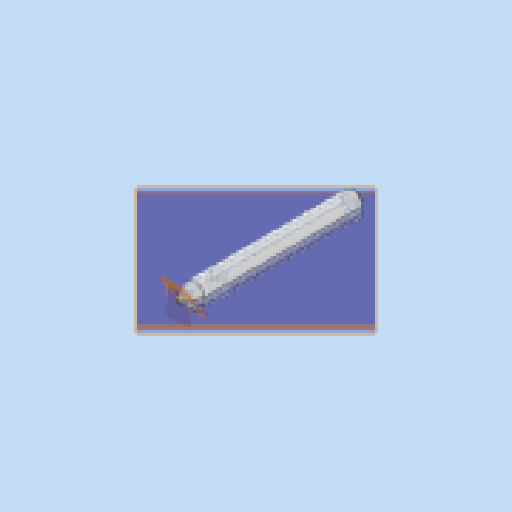
# Autodesk Inventor part: Shell
Saved by Autodesk Inventor 2024 (Build 280153000, 153)
## iProperties
Created: 2025-03-21
Part Number: Shell
Material: Generic
Document SubType Name: Modeling
Designer: XxPan
Density: 1 g/cm^3
Appearance: Default
Author: XxPan
Autodesk Inventor part; units mm, degrees
ref_plane "YZ Plane" through (0, 0, 0) normal (1, 0, 0) x (0, 1, 0)
ref_plane "XZ Plane" through (0, 0, 0) normal (0, 1, 0) x (-1, 0, 0)
sketch "Sketch1" plane through (0, 0, 0) normal (0, 0, 1) x (1, 0, 0)
  line L0 (0, 0) -> (0, -6) construction
  line L1 (-9, 0) -> (-9, -6)
  line L2 (9, -6) -> (9, 0)
  arc A0 (9, 0) -> (-9, 0) centre (0, 0) ccw
  arc A1 (-9, -6) -> (9, -6) centre (0, -6) ccw
  point P0 (0, -3)
  dimension "d0" = 6
  dimension "d1" = 18
  constraints: 8 end point, 4 point on circle, 4 tangent, 2 centre point, 1 midpoint, 1 parallel, 1 vertical
  measures "d0" distance of L0.start L0.end
  measures "d1" diameter of A1
extrude "Extrusion1" add sketch "Sketch1" against normal blind 150
chamfer "Chamfer1" distance 2 angle 45 4 edges at (0, 9, -150) (9, -3, -150) (0, -15, -150) (-9, -3, -150)
shell "Shell1" thickness 1 removed faces 1 at (1.0638, -8.805, 0)
ref_plane "Work Plane1" through (0, 0, 15) normal (0, 0, 1) x (1, 0, 0)
sketch "Sketch2" plane through (0, 0, 15) normal (0, 0, 1) x (1, 0, 0)
  circle A0 centre (0, 0) radius 2
  dimension "d3" = 4
  constraints: 1 centre point, 1 coincident
  measures "d3" diameter of A0
loft "Loft1" add profiles "Sketch1", "Sketch2" separate body
sketch "Sketch3" plane through (0, 0, 15) normal (0, 0, 1) x (1, 0, 0)
  circle A0 centre (0, 0) radius 0.6
  dimension "d14" = 1.2
  constraints: 1 centre point, 1 coincident
  measures "d14" diameter of A0
ref_plane "Work Plane2" through (-8.2598, -14.025, 0) normal (0, 0, 1) x (1, 0, 0)
extrude "Extrusion2" cut sketch "Sketch3" against normal up to surface (15 mm away) bodies 2
sketch "Sketch4" plane through (0, 0, 0) normal (1, 0, 0) x (0, 1, 0)
  line L0 (-6, 0) -> (-15, 0) projected
  line L1 (-15, 0) -> (14.5608, 20.6987)
  line L2 (-15, 0) -> (21.0871, 0) construction
  point P0 (0, 0)
  dimension "d17" = 35
  constraints: 4 end point, 1 equal length, 1 horizontal
  measures "d17" angle of L2 L1
surface extrude "ExtrusionSrf1" sketch "Sketch4" along normal mid plane 20 shown yes curves L1
sketch "Sketch5" plane through (0, 0, 15) normal (0, 0, 1) x (1, 0, 0)
  circle A0 centre (0, -7) radius 4
  line L0 (0, -18) -> (0, 3) construction
  line L1 (10, -15) -> (-10, -15) projected
  line L2 (-4, -7) -> (-4, -15)
  line L3 (4, -7) -> (4, -15)
  point P0 (0, 0)
  dimension "d20" = 8
  dimension "d21" = 8
  constraints: 4 end point, 3 point on line, 2 perpendicular, 2 point on circle, 2 tangent, 1 centre point
  measures "d20" diameter of A0
  measures "d21" distance from line of L1 A0.centre
extrude "Extrusion3" cut sketch "Sketch5" against normal up to surface surface through (0, -15, 0) normal (0, 0.5735764, -0.819152) bodies 2
ref_plane "Work Plane4" through (-10, 15.7079, 19.0604) normal (0, -0.5735764, 0.819152) x (1, 0, 0)
sketch "Sketch6" plane through (0, 0, 0) normal (0, 0, 1) x (1, 0, 0)
  arc A0 (4, -7) -> (-4, -7) centre (0, -7) ccw projected
  circle A1 centre (0, -7) radius 4
  point P0 (0, 0)
  point P1 (4, -7)
  constraints: 1 coincident, 3 other
extrude "Extrusion4" cut sketch "Sketch6" along normal up to surface surface through (0, -15, 0) normal (0, 0.5735764, -0.819152) bodies 2
sketch "Sketch7" plane through (4, -12.3169, 1.8787) normal (0, -0.5735764, 0.819152) x (1, 0, 0)
  line L0 (-4, 7.3739) -> (-4, 3.3739) construction
  line L1 (-8, 7.3739) -> (-8, 3.3739)
  line L2 (0, 3.3739) -> (0, 7.3739)
  arc A0 (0, 7.3739) -> (-8, 7.3739) centre (-4, 7.3739) ccw
  arc A1 (-8, 3.3739) -> (0, 3.3739) centre (-4, 3.3739) ccw
  line L3 (0, 0) -> (0, 6.4908) projected
  ellipse E0 centre (-4, 6.4908) end of major axis (-4, 1.6077) minor radius 4 (0, 6.4908) -> (-8, 6.4908) ccw projected
  point P0 (-4, 9.0119)
  point P1 (-4, 5.3739)
  point P2 (0, 6.4908)
  dimension "d27" = 4
  dimension "d28" = 8
  constraints: 8 end point, 4 point on circle, 4 tangent, 2 centre point, 1 collinear, 1 midpoint, 1 parallel, 1 vertical, 2 other
  measures "d27" distance of L0.start L0.end
  measures "d28" diameter of A1
extrude "Extrusion5" cut sketch "Sketch7" along normal blind 1 and the other way blind 1 contours E0 L2 A1 L1 bodies 2
ref_plane "Work Plane5" through (5, -1.8, -20.16) normal (0, 0, -1) x (-1, 0, 0)
sketch "Sketch8" plane through (5, -1.8, -20.16) normal (0, 0, -1) x (-1, 0, 0)
  arc A0 (13, 1.8) -> (-3, 1.8) centre (5, 1.8) ccw projected
  line L0 (-3, 1.8) -> (-3, -4.2) projected
  line L1 (13, -4.2) -> (13, 1.8) projected
  arc A1 (-3, -4.2) -> (13, -4.2) centre (5, -4.2) ccw projected
  line L2 (-1, 7.0915) -> (-1, -4.2)
  line L3 (-3, -4.2) -> (-1, -2.2)
  line L4 (-3, -4.2) -> (-0.1716, -4.2) construction
  dimension "d33" = 2
  dimension "d34" = 45
  constraints: 6 end point, 1 equal length, 1 horizontal, 1 parallel, 1 point on circle, 1 point on line
  measures "d33" distance between parallel lines of L0 L2
  measures "d34" angle of L4 L3
extrude "Extrusion6" add sketch "Sketch8" along normal blind 3 contours L1 A1 L3 L2 A0 bodies 1
sketch "Sketch9" plane through (5, -1.8, -20.16) normal (0, 0, 1) x (1, 0, 0)
  circle A0 centre (-5, 2) radius 1.5 projected
  line L0 (-3.9393, 3.0607) -> (-5, 4.1213)
  line L1 (-5, 4.1213) -> (-6.0607, 3.0607)
  point P0 (-5, 1.8)
  constraints: 4 end point, 2 point on circle, 2 tangent, 1 perpendicular, 1 vertical alignment
extrude "Extrusion7" cut sketch "Sketch9" against normal up to surface (3 mm away) bodies 1
ref_plane "Work Plane8" through (9, -3, -148) normal (0, -1, 0) x (-0.7071068, 0, -0.7071068)
ref_plane "Work Plane6" through (9, 0, -148) normal (0, -1, 0) x (-0.7071068, 0, -0.7071068)
ref_plane "Work Plane7" through (9, -6, -148) normal (0, -1, 0) x (-0.7071068, 0, -0.7071068)
sketch "Sketch10" plane through (0, 0, -150) normal (0, 0, -1) x (-1, 0, 0)
  arc A0 (-1.625, -5.875) -> (1.625, -5.875) centre (0, -5.875) ccw construction
  line L0 (-1.625, -0.125) -> (-1.625, -5.875) construction
  line L1 (1.625, -5.875) -> (1.625, -0.125) construction
  arc A1 (1.625, -0.125) -> (-1.625, -0.125) centre (0, -0.125) ccw construction
  line L2 (-1.825, -0.125) -> (-1.825, -5.875)
  arc A2 (-1.825, -5.875) -> (1.825, -5.875) centre (0, -5.875) ccw
  line L3 (1.825, -5.875) -> (1.825, -0.125)
  arc A3 (1.825, -0.125) -> (-1.825, -0.125) centre (0, -0.125) ccw
  point P0 (0, 0)
  dimension "d0" = 6
  dimension "d1" = 18
  dimension "d14" = 1.2
  dimension "d39" = 0.2
  constraints: 4 end point, 4 point on circle, 2 centre point, 3 other
  measures "d39" radial gap between concentric circles of A1 A3
extrude "Extrusion8" cut sketch "Sketch10" against normal up to surface (1 mm away) bodies 1
body "Solid1"
body "Solid2"
body "Srf1"
